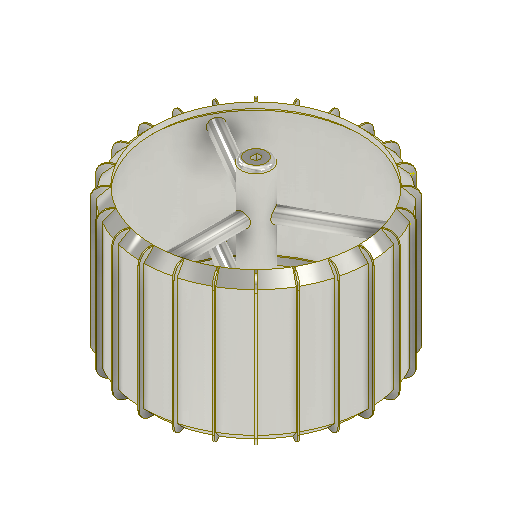
# Autodesk Inventor part: DébutRoue_Inventor
Saved by Autodesk Inventor 2025 (Build 290162010, 162A)
## iProperties
Created: 2024-07-23
Part Number: DébutRoue_Inventor
Material: Générique
Document SubType Name: Modeling
Designer: damie
Density: 1 g/cm^3
Appearance: Argent
Author: damie
Autodesk Inventor part; units mm, degrees
ref_plane "YZ Plane" through (0, 0, 0) normal (1, 0, 0) x (0, 1, 0)
sketch "Esquisse1" plane through (0, 0, 0) normal (0, 1, 0) x (-1, 0, 0)
  circle A0 centre (0, 0) radius 70
  circle A1 centre (0, 0) radius 77
  dimension "d0" = 7
  dimension "d1" = 154
  constraints: 2 centre point, 2 coincident
  measures "d0" radial gap between concentric circles of A1 A0
  measures "d1" diameter of A1
extrude "Extrusion1" add sketch "Esquisse1" along normal blind 100
chamfer "Chanfrein1" distance 7 angle 45 1 edges at (77, 0, 0)
chamfer "Chanfrein2" distance 7 angle 45 1 edges at (77, 100, 0)
sketch "Esquisse2" plane through (0, 0, 0) normal (0, 1, 0) x (-1, 0, 0)
  line L0 (0.5, -80) -> (-0.5, -80)
  line L1 (-0.5, -80) -> (-0.5, -70)
  line L2 (-0.5, -70) -> (0.5, -70)
  line L3 (0.5, -70) -> (0.5, -80)
  point P0 (0, 0)
  point P1 (0, -80)
  dimension "d10" = 10
  dimension "d11" = 70
  dimension "d12" = 1
  dimension "d13" = 0.5
  constraints: 8 end point, 2 parallel, 1 horizontal, 1 midpoint, 1 perpendicular
  measures "d10" distance from line of L2 point (0, -80)
  measures "d11" distance from line of point (0, 0) L2
  measures "d12" distance of L0.start L0.end
  measures "d13" distance from line of point (0, 0) L3
extrude "Extrusion2" add sketch "Esquisse2" along normal blind 100
fillet "Congé1" radius 7 2 edges at (0, 0, -80) (0, 100, -80)
pattern_circular "Réseau circulaire1" count 24 over 360 about axis through (0, -10, 0) along (0, 1, 0) of "Extrusion2", "Congé1"
ref_plane "Plan tangent roue" through (66.4326, 7, -38.9322) normal (-0.7934, 0, 0.6088) x (-0.132, 0.9762, -0.1721)
sketch "Esquisse3" plane through (66.4326, 7, -38.9322) normal (-0.7934, 0, 0.6088) x (-0.132, 0.9762, -0.1721)
  circle A0 centre (44.0487, 0) radius 5
  circle A1 centre (20.746, 0) radius 2.5
  circle A2 centre (22.9388, 9.8685) radius 2.5
  circle A3 centre (65.1587, -9.8685) radius 2.5
  circle A4 centre (67.3515, 0) radius 2.5
  line L0 (-6.6335, 2.4097) -> (0, 0) projected
  line L1 (83.9525, -18.6542) -> (88.0974, 0) projected
  line L2 (0, 0) -> (88.0974, 0) construction
  line L3 (4.145, 18.6542) -> (-2.8848, 19.2805) projected
  line L4 (4.145, 18.6542) -> (83.9525, -18.6542) construction
  line L5 (4.145, 18.6542) -> (88.0974, 0) projected
  line L6 (83.9525, -18.6542) -> (0, 0) projected
  point P0 (-4.7609, 10.8455)
  dimension "d20" = 5
  dimension "d21" = 5
  dimension "d22" = 5
  dimension "d23" = 5
  dimension "d24" = 10
  dimension "d25" = 4.5
  dimension "d26" = 4.5
  dimension "d27" = 4.5
  dimension "d28" = 4.5
  constraints: 5 centre point, 4 end point, 4 point on line, 1 horizontal, 1 midpoint
  measures "d20" diameter of A1
  measures "d21" diameter of A3
  measures "d22" diameter of A4
  measures "d23" diameter of A2
  measures "d24" diameter of A0
  measures "d25" distance from line of L5 A2.centre
  measures "d26" distance from line of A4.centre L5
  measures "d27" distance from line of L6 A3.centre
  measures "d28" distance from line of L6 A1.centre
extrude "Extrusion3" [suppressed]
pattern_circular "Réseau circulaire2" [suppressed]
ref_plane "Plan ce" through (0, 7, 0) normal (0, 1, 0) x (-1, 0, 0)
sketch "Esquisse5" plane through (0, 7, 0) normal (0, 1, 0) x (-1, 0, 0)
  circle A0 centre (0, 0) radius 74
  dimension "d36" = 148
  constraints: 1 centre point, 1 coincident
  measures "d36" diameter of A0
extrude "Extrusion4" cut sketch "Esquisse5" along normal blind 86
chamfer "Chanfrein3" distance 3 angle 45 1 edges at (70, 93, 0)
chamfer "Chanfrein4" distance 3 angle 45 1 edges at (70, 7, 0)
sketch "Esquisse7" plane through (0, 7, 0) normal (0, 1, 0) x (-1, 0, 0)
  circle A0 centre (0, 0) radius 10
  dimension "d45" = 20
  constraints: 1 centre point, 1 coincident
  measures "d45" diameter of A0
extrude "Extrusion5" add sketch "Esquisse7" along normal blind 110
sketch "Esquisse8" plane through (0, 0, 0) normal (0, 0, 1) x (1, 0, 0)
  circle A0 centre (0, 15) radius 5
  line L0 (0.5, 0) -> (-0.5, 0) projected
  circle A1 centre (0, 85) radius 5
  point P0 (0, 0)
  point P1 (0, 0)
  dimension "d48" = 10
  dimension "d49" = 15
  dimension "d55" = 10
  dimension "d56" = 70
  constraints: 2 centre point, 1 midpoint
  measures "d48" diameter of A0
  measures "d49" distance of A0.centre point (0, 0)
  measures "d55" diameter of A1
  measures "d56" distance of A0.centre A1.centre
extrude "Extrusion6" add sketch "Esquisse8" along normal blind 76
pattern_circular "Réseau circulaire3" count 3 over 360 about axis through (0, -10, 0) along (0, 1, 0) of "Extrusion6"
sketch "Schizzo9" plane through (0, 117, 0) normal (0, 1, 0) x (1, 0, 0)
  arc A0 (-1.8743, -2.125) -> (-1.8743, 2.125) centre (0, 0) ccw
  line L0 (-1.8743, -2.125) -> (-1.8743, 2.125)
  point P0 (-1.8743, 0)
  dimension "d57" = 5.667
  dimension "d58" = 4.25
  dimension "d62" = 1.8743
  constraints: 2 end point, 2 point on circle, 1 centre point, 1 coincident, 1 midpoint, 1 vertical
  measures "d57" diameter of A0
  measures "d58" distance of L0.start L0.end
  measures "d62" distance of point (0, 0) point (-1.874, 0)
extrude "Estrusione7" cut sketch "Schizzo9" against normal blind 10.67
fillet "Raccordo2" radius 3 1 edges at (10, 117, 0)
